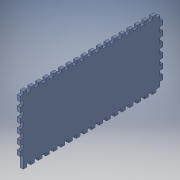
# Autodesk Inventor part: 000.202 - Боковая стенка пустая
Saved by Autodesk Inventor 2019 (Build 230136000, 136)
## iProperties
Created: 2020-02-27
Part Number: 000.202 - Боковая стенка пустая
Material: Пластик АБС
Document SubType Name: Modeling
Designer: Петров Иван
Density: 1.06 g/cm^3
Appearance: Резина — синяя
Author: Петров Иван
Autodesk Inventor part; units mm, degrees
ref_plane "YZ Plane" through (0, 0, 0) normal (1, 0, 0) x (0, 1, 0)
ref_plane "XZ Plane" through (0, 0, 0) normal (0, 1, 0) x (-1, 0, 0)
ref_plane "XY Plane" through (0, 0, 0) normal (0, 0, 1) x (1, 0, 0)
sketch "Эскиз1" plane through (0, 0, 0) normal (1, 0, 0) x (0, 1, 0)
  line L0 (-32.5, 72) -> (32.5, 72)
  line L1 (32.5, 72) -> (32.5, -72)
  line L2 (32.5, -72) -> (-32.5, -72)
  line L3 (-32.5, -72) -> (-32.5, 72)
  line L4 (-32.5, 72) -> (32.5, -72) construction
  line L5 (32.5, 72) -> (-32.5, -72) construction
  point P0 (0, 0)
  dimension "d0" = 65
  dimension "d1" = 144
  constraints: 12 end point, 2 midpoint, 2 parallel, 1 horizontal, 1 perpendicular
  measures "d0" distance of L1.end L2.end
  measures "d1" distance of L0.end L1.end
extrude "Выдавливание1" add sketch "Эскиз1" along normal blind 3
sketch "Эскиз2" plane through (3, 0, 0) normal (1, 0, 0) x (0, 0, -1)
  line L0 (-72, -32.5) -> (72, -32.5) projected
  line L1 (-72, -32.5) -> (-68, -32.5)
  line L2 (-68, -32.5) -> (-68, -35.5)
  line L3 (-68, -35.5) -> (-72, -35.5)
  line L4 (-72, -35.5) -> (-72, -32.5)
  point P0 (0, 0)
  dimension "d4" = 4
  dimension "d5" = 3
  constraints: 8 end point, 2 parallel, 1 horizontal, 1 perpendicular
  measures "d4" distance of L2.end L3.end
  measures "d5" distance of L1.end L2.end
extrude "Выдавливание2" add sketch "Эскиз2" against normal blind 3
pattern_linear "Прямоуг.массив1" count 18 spacing 8 along (0, 0, -1) of "Выдавливание2"
sketch "Эскиз3" plane through (3, 0, 0) normal (1, 0, 0) x (0, 0, -1)
  line L0 (72, 32.5) -> (-72, 32.5) projected
  line L1 (-72, 32.5) -> (-75, 32.5)
  line L2 (-75, 32.5) -> (-75, 27.5)
  line L3 (-75, 27.5) -> (-72, 27.5)
  line L4 (-72, 27.5) -> (-72, 32.5)
  line L5 (72, -32.5) -> (72, 32.5) projected
  line L6 (72, 27.5) -> (75, 27.5)
  line L7 (75, 27.5) -> (75, 22.5)
  line L8 (75, 22.5) -> (72, 22.5)
  line L9 (72, 22.5) -> (72, 27.5)
  point P0 (0, 0)
  dimension "d11" = 3
  dimension "d12" = 5
  dimension "d13" = 3
  dimension "d14" = 5
  dimension "d15" = 5
  constraints: 16 end point, 4 parallel, 2 horizontal, 2 perpendicular, 1 point on line
  measures "d11" distance of L3.end L2.end
  measures "d12" distance of L2.end L1.end
  measures "d13" distance of L7.end L8.end
  measures "d14" distance of L6.end L7.end
  measures "d15" distance between parallel lines of L0 L6
extrude "Выдавливание3" add sketch "Эскиз3" against normal blind 3
pattern_linear "Прямоуг.массив2" count 6 spacing 10 along (0, -1, 0) of "Выдавливание3"
mirror "Зеркальное отражение1" about plane through (0, 0, 0) normal (0, 1, 0) of "Выдавливание2", "Прямоуг.массив1"
sketch "Эскиз4" plane through (0, 0, 0) normal (-1, 0, 0) x (0, 0, 1)
  line L0 (-24.49, 2.034) -> (-35.69, 2.034) projected
  line L1 (-24.49, 2.034) -> (-24.49, -7.766) projected
  line L2 (-35.69, 2.034) -> (-35.69, -7.766) projected
  line L3 (-35.69, -8.166) -> (-24.49, -8.166) projected
  line L4 (-35.69, -7.766) -> (-35.69, -8.166) projected
  line L5 (-24.49, -8.166) -> (-24.49, -7.766) projected
  line L6 (34.27, -8.7) -> (18.25, -8.7) projected
  line L7 (18.25, -8.7) -> (18.25, 6.6) projected
  line L8 (34.27, 6.6) -> (18.25, 6.6) projected
  line L9 (34.27, -8.7) -> (34.27, 6.6) projected
  line L10 (38.35, 6.5) -> (38.35, -8.7) projected
  line L11 (51.25, 6.5) -> (38.75, 6.5) projected
  line L12 (69.65, -8.7) -> (69.65, 6.5) projected
  line L13 (38.35, 6.5) -> (69.65, 6.5)
  line L14 (69.65, 6.5) -> (69.65, -8.7)
  line L15 (69.65, -8.7) -> (38.35, -8.7)
  line L16 (38.35, -8.7) -> (38.35, 6.5)
  point P0 (0, 0)
  dimension "d23" = 0
  constraints: 8 end point, 2 parallel, 1 horizontal, 1 perpendicular
  measures "d23" distance between parallel lines of L12 L14
extrude "Выдавливание4" [suppressed]
sketch "Эскиз5" plane through (3, 35.5, -64) normal (0, 1, 0) x (1, 0, 0)
  line L0 (0, 4) -> (0, 8) projected
  line L1 (-3, -56) -> (-3, -60) projected
  line L2 (0, 4) -> (-3, 4)
  line L3 (-3, 4) -> (-3, -56)
  line L4 (-3, -56) -> (0, -56)
  line L5 (0, -56) -> (0, 4)
  point P0 (-3, -64)
  constraints: 8 end point, 2 parallel, 1 horizontal, 1 perpendicular
extrude "Выдавливание5" [suppressed]
